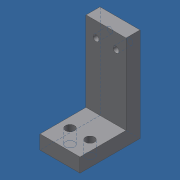
# Autodesk Inventor part: EndSwitchBracket
Saved by Autodesk Inventor 2021 (Build 250183000, 183)
## iProperties
Created: 2022-09-08
Part Number: EndSwitchBracket
Material: Generic
Document SubType Name: Modeling
Designer: Nathann
Density: 1 g/cm^3
Appearance: Default
Author: Nathann
Autodesk Inventor part; units mm, degrees
ref_plane "YZ Plane" through (0, 0, 0) normal (1, 0, 0) x (0, 1, 0)
ref_plane "XZ Plane" through (0, 0, 0) normal (0, 1, 0) x (-1, 0, 0)
ref_plane "XY Plane" through (0, 0, 0) normal (0, 0, 1) x (1, 0, 0)
sketch "Sketch1" plane through (0, 0, 0) normal (0, 0, 1) x (1, 0, 0)
  circle A0 centre (-5, 3.0188) radius 1.5
  circle A1 centre (-15, 3.0188) radius 1.5
  line L0 (0, -36.4812) -> (-20, -36.4812)
  line L1 (-20, -36.4812) -> (-20, 10.5188)
  line L2 (-20, 10.5188) -> (0, 10.5188)
  line L3 (0, 10.5188) -> (0, -36.4812)
  dimension "d0" = 3
  dimension "d1" = 3
  dimension "d2" = 10
  dimension "d3" = 20
  dimension "d4" = 7.5
  dimension "d5" = 7.5
  dimension "d6" = 5
  dimension "d7" = 47
  constraints: 8 end point, 2 centre point, 2 parallel, 1 horizontal, 1 perpendicular
  measures "d0" diameter of A0
  measures "d1" diameter of A1
  measures "d2" distance of A0.centre A1.centre
  measures "d3" distance of L1.end L2.end
  measures "d4" distance from line of L2 A0.centre
  measures "d5" distance from line of L2 A1.centre
  measures "d6" distance from line of L3 A0.centre
  measures "d7" distance of L2.end L0.start
extrude "Extrusion1" add sketch "Sketch1" along normal blind 7
sketch "Sketch2" plane through (-20, -36.4812, 0) normal (0, -1, 0) x (1, 0, 0)
  line L0 (0, 0) -> (0, 7) projected
  line L1 (0, 0) -> (20, 0)
  line L2 (20, 0) -> (20, 30)
  line L3 (20, 30) -> (0, 30)
  line L4 (0, 30) -> (0, 0)
  circle A0 centre (15, 20) radius 2.25
  circle A1 centre (5, 20) radius 2.25
  dimension "d10" = 30
  dimension "d11" = 4.5
  dimension "d12" = 4.5
  dimension "d13" = 10
  dimension "d14" = 5
  dimension "d15" = 10
  constraints: 8 end point, 2 centre point, 2 parallel, 1 horizontal, 1 perpendicular
  measures "d10" distance of L1.end L2.end
  measures "d11" diameter of A0
  measures "d12" diameter of A1
  measures "d13" distance of A1.centre A0.centre
  measures "d14" distance from line of L2 A0.centre
  measures "d15" distance from line of L3 A0.centre
extrude "Extrusion2" add sketch "Sketch2" against normal blind 7
equation "\"d5\" = d4"
equation "\"d12\" = d11"
body "Solid1"
